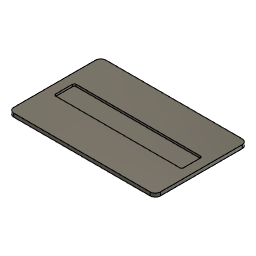
RFID CARD (Autodesk Fusion 360 design; units mm, degrees)
Autodesk Fusion 360 part; units mm, degrees
sketch "Skizze1" plane through (0, 0, 0) normal (0, 1, 0) x (1, 0, 0)
  line L0 (43, 27) -> (-43, 27)
  line L1 (-43, 27) -> (-43, -27)
  line L2 (-43, -27) -> (43, -27)
  line L3 (43, -27) -> (43, 27)
  line L4 (43, 27) -> (-43, -27) construction
  line L5 (-43, 27) -> (43, -27) construction
  dimension "d1" = 54
  dimension "d2" = 86
  constraint horizontal L0
  constraint perpendicular L0 L1
  constraint parallel L0 L2
  constraint parallel L1 L3
  constraint coincident L4 origin
  constraint coincident L5 origin
  measures "d1" distance of L0.end L1.end
  measures "d2" distance of L0.start L0.end
extrude "Extrusion1" add sketch "Skizze1" along normal blind 2
fillet "Abrundung1" radius 3 4 edges at (43, 1, -27) (43, 1, 27) (-43, 1, 27) (-43, 1, -27)
sketch "Skizze2" plane through (0, 2, 0) normal (0, 1, 0) x (-1, 0, 0)
  arc A0 (40, -27) -> (43, -24) centre (40, -24) ccw
  line L0 (43, -24) -> (43, 24)
  arc A1 (43, 24) -> (40, 27) centre (40, 24) ccw
  line L1 (40, 27) -> (-40, 27)
  arc A2 (-40, 27) -> (-43, 24) centre (-40, 24) ccw
  line L2 (-43, 24) -> (-43, -24)
  arc A3 (-43, -24) -> (-40, -27) centre (-40, -24) ccw
  line L3 (-40, -27) -> (40, -27)
  line L4 (37.5, -6) -> (-37.5, -6)
  line L5 (-37.5, -6) -> (-37.5, 6)
  line L6 (-37.5, 6) -> (37.5, 6)
  line L7 (37.5, 6) -> (37.5, -6)
  line L8 (37.5, -6) -> (-37.5, 6) construction
  line L9 (-37.5, -6) -> (37.5, 6) construction
  dimension "d7" = 12
  dimension "d8" = 75
  constraint horizontal L4
  constraint perpendicular L4 L5
  constraint parallel L4 L6
  constraint parallel L5 L7
  constraint coincident L8 origin
  constraint coincident L9 origin
  measures "d7" distance of L4.end L5.end
  measures "d8" distance of L4.start L4.end
extrude "Extrusion2" cut sketch "Skizze2" against normal blind 1.2 contours L4 L5 L6 L7
fillet "Abrundung2" radius 1 4 edges at (37.5, 1.4, -6) (37.5, 1.4, 6) (-37.5, 1.4, -6) (-37.5, 1.4, 6)
